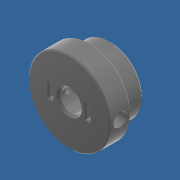
# Autodesk Inventor part: Print_Parts_A1
Saved by Autodesk Inventor 2020 (Build 240168000, 168)
## iProperties
Created: 2020-10-05
Part Number: Print_Parts_A1
Material: PC/ABS プラスチック
Document SubType Name: Modeling
Designer: kenta iguchi
Density: 0.357273 g/cm^3
Appearance: 滑らか - 黒
Author: kenta iguchi
Autodesk Inventor part; units mm, degrees
ref_plane "XZ Plane" through (0, 0, 0) normal (0, 1, 0) x (-1, 0, 0)
ref_plane "XY Plane" through (0, 0, 0) normal (0, 0, 1) x (1, 0, 0)
sketch "スケッチ1" plane through (0, 0, 0) normal (0, 0, 1) x (1, 0, 0)
  circle A0 centre (0, 0) radius 15.6
  dimension "d0" = 31.2
  constraints: 1 centre point, 1 coincident
  measures "d0" diameter of A0
extrude "押し出し1" add sketch "スケッチ1" along normal blind 10
sketch "スケッチ2" plane through (0, 0, 10) normal (0, 0, 1) x (1, 0, 0)
  circle A0 centre (0, 0) radius 15.6 projected
  circle A1 centre (0, 0) radius 19.5
  dimension "d3" = 39
  constraints: 1 centre point, 1 coincident
  measures "d3" diameter of A1
extrude "押し出し2" add sketch "スケッチ2" along normal blind 10 contours A0 | A1
chamfer "面取り1" distance 1 angle 45 1 edges at (-15.6, 0, 0)
chamfer "面取り2" distance 0.5 angle 45 2 edges at (-19.5, 0, 20) (-19.5, 0, 10)
sketch "スケッチ3" plane through (0, 0, 20) normal (0, 0, 1) x (1, 0, 0)
  circle A0 centre (0, 0) radius 19 projected
  circle A1 centre (0, 0) radius 5.1
  dimension "d12" = 10.2
  constraints: 1 centre point, 1 coincident
  measures "d12" diameter of A1
extrude "押し出し3" cut sketch "スケッチ3" against normal through all contours A1
chamfer "面取り3" distance 1 angle 45 1 edges at (-5.1, 0, 20)
ref_plane "作業平面1" through (20, 0, 0) normal (1, 0, 0) x (0, 1, 0)
sketch "スケッチ4" plane through (20, 0, 0) normal (1, 0, 0) x (0, 1, 0)
  line L0 (19.5, 19.5) -> (-19.5, 19.5) projected
  line L1 (-19.5, 10.5) -> (19.5, 10.5) projected
  line L2 (-19, 20) -> (19, 20) projected
  point P0 (0, 0)
  point P1 (0, 15)
  dimension "d44" = 5
  measures "d44" distance from line of point (0, 15) L2
hole "穴1" at (20, 0, 15) direction (-1, 0, 0) diameter 3.3 depth 17.75 tip angle 118
sketch "スケッチ5" plane through (20, 0, 0) normal (1, 0, 0) x (0, 1, 0)
  line L0 (-19.5, 10.5) -> (19.5, 10.5) projected
  line L1 (19.5, 19.5) -> (-19.5, 19.5) projected
  line L2 (-19, 20) -> (19, 20) projected
  point P0 (0, 0)
  point P1 (1.65, 15)
  point P2 (0, 15)
  point P3 (-1.65, 15)
  point P4 (1.65, 15)
  dimension "d45" = 5
  constraints: 1 vertical alignment, 3 other
  measures "d45" distance from line of point (0, 15) L2
hole "穴2" at (20, 0, 15) direction (-1, 0, 0) diameter 6.5 depth 5
sketch "スケッチ6" plane through (0, 0, 20) normal (0, 0, 1) x (1, 0, 0)
  circle A0 centre (0, 0) radius 19 projected
  line L0 (8, 3.15) -> (9.8, 3.15)
  line L1 (9.8, 3.15) -> (9.8, -3.15)
  line L2 (9.8, -3.15) -> (8, -3.15)
  line L3 (8, -3.15) -> (8, 3.15)
  dimension "d34" = 1.8
  dimension "d35" = 6.3
  dimension "d36" = 3.15
  dimension "d37" = 8
  constraints: 8 end point, 2 parallel, 1 horizontal, 1 perpendicular
  measures "d34" distance of L1.end L2.end
  measures "d35" distance of L0.end L1.end
  measures "d36" distance from line of L2 A0.centre
  measures "d37" distance from line of L3 A0.centre
extrude "押し出し4" cut sketch "スケッチ6" against normal blind 8.5 contours L0 L1 L2 L3
mirror "ミラー1" about plane through (0, 0, 0) normal (1, 0, 0) of "穴2", "穴1", "押し出し4"
chamfer "面取り4" distance 2 angle 45 1 edges at (-5.1, 0, 0)
chamfer "面取り5" distance 0.5 angle 45 8 edges at (9.8, 0, 20) (8, 0, 20) (8.9, -3.15, 20) (8.9, 3.15, 20) (-8.9, 3.15, 20) (-8.9, -3.15, 20) (-9.8, 0, 20) (-8, 0, 20)
